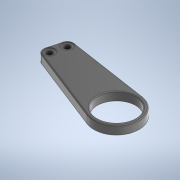
# Autodesk Inventor part: RearBumper
Saved by Autodesk Inventor 2020 (Build 240168000, 168)
## iProperties
Part Number: RearBumper
Material: PC/ABS プラスチック
Document SubType Name: Modeling
Designer: Masato Kubotera
Density: 0.357273 g/cm^3
Appearance: 滑らか - 黒
Description: TPU
Author: Masato Kubotera
Autodesk Inventor part; units mm, degrees
ref_plane "YZ Plane" through (0, 0, 0) normal (1, 0, 0) x (0, 1, 0)
ref_plane "XZ Plane" through (0, 0, 0) normal (0, 1, 0) x (-1, 0, 0)
ref_plane "XY Plane" through (0, 0, 0) normal (0, 0, 1) x (1, 0, 0)
derived "Trunk_basis.ipt"
sketch "スケッチ1" plane through (0, 0, 0) normal (0, 1, 0) x (-1, 0, 0)
  line L0 (0, 22) -> (0, -142.9) construction
  circle A0 centre (5, 0) radius 10.5 construction
  line L1 (-7, 16) -> (36, 16) construction
  line L2 (36, 16) -> (36, -16) construction
  line L3 (36, -16) -> (-7, -16) construction
  line L4 (-7, -16) -> (-7, 16) construction
  line L5 (-7, 16) -> (36, -16) construction
  line L6 (36, 16) -> (-7, -16) construction
  line L7 (33, 13.5) -> (6, 13.5) construction
  line L8 (6, 13.5) -> (6, -13.5) construction
  line L9 (6, -13.5) -> (33, -13.5) construction
  line L10 (33, -13.5) -> (33, 13.5) construction
  line L11 (33, 13.5) -> (6, -13.5) construction
  line L12 (6, 13.5) -> (33, -13.5) construction
  line L13 (-7, 0) -> (36, 0) construction
  arc A1 (5, 16) -> (-7, 10.583) centre (5, 0) ccw construction
  line L14 (43.75, -16.25) -> (5, -16.25)
  line L15 (5, 16.25) -> (43.75, 16.25)
  line L16 (44.75, 15.25) -> (44.75, -15.25)
  arc A2 (5, 16.25) -> (-6.7376, 11.2379) centre (5, 0) ccw
  arc A3 (-6.7376, 11.2379) -> (-7.25, 9.9174) centre (-6.2711, 10.2972) ccw
  circle A4 centre (6, 13.5) radius 1.35
  line L17 (19.5, 13.5) -> (19.5, -13.5) construction
  circle A5 centre (33, 13.5) radius 1.35
  line L18 (-15, 22) -> (-20, 17)
  line L19 (-20, 17) -> (-20, -19)
  line L20 (-20, -19) -> (-28.5, -27.5)
  line L21 (-28.5, -27.5) -> (-28.5, -103)
  line L22 (57.5, -22.5) -> (57.5, 17)
  line L23 (57.5, 17) -> (52.5, 22)
  line L24 (52.5, 22) -> (-15, 22)
  line L25 (-35.5597, -116.5529) -> (-28.5, -142.9)
  line L26 (-16, -139) -> (-16, -94) construction
  line L27 (-7.5, -140.4849) -> (-7.5, -142.9)
  line L28 (-7.5, -142.9) -> (7.5, -142.9)
  line L29 (7.5, -140.4849) -> (7.5, -142.9)
  arc A6 (-7.5, -140.4849) -> (-8.9849, -139) centre (-8.2425, -139.7425) ccw
  line L30 (-17.5, -138.9955) -> (-17.5, -133) construction
  line L31 (-19, -133) -> (-16, -133) construction
  line L32 (-19, -133) -> (-19, -139) construction
  line L33 (-16, -133) -> (-16, -139) construction
  line L34 (-15, 22) -> (-10, 22) construction
  line L35 (-10, 22) -> (-10, -22) construction
  line L36 (-10, -22) -> (-15, -22) construction
  line L37 (-15, -22) -> (-15, 22) construction
  line L38 (-15, 22) -> (-10, -22) construction
  line L39 (-10, 22) -> (-15, -22) construction
  line L40 (-12.5, 22) -> (-12.5, -22) construction
  line L41 (-10, 0) -> (-15, 0) construction
  circle A7 centre (-12.5, 17.75) radius 1.6
  line L42 (-15, 10) -> (-12.5, 10) construction
  line L43 (-12.5, 10) -> (-12.5, -10) construction
  line L44 (-12.5, -10) -> (-15, -10) construction
  line L45 (-15, -10) -> (-15, 10) construction
  line L46 (-15, 10) -> (-12.5, -10) construction
  line L47 (-12.5, 10) -> (-15, -10) construction
  line L48 (-12.25, 10.25) -> (-15.25, 10.25)
  line L49 (-15.25, 8.15) -> (-15.25, -8.15)
  line L50 (-15.25, -10.25) -> (-12.25, -10.25)
  line L51 (-12.25, -8.15) -> (-12.25, 8.15)
  line L52 (-12.25, 10.25) -> (-15.25, -10.25) construction
  line L53 (-15.25, 10.25) -> (-12.25, -10.25) construction
  arc A8 (-15.25, 10.25) -> (-15.25, 8.15) centre (-15.25, 9.2) ccw
  line L54 (-13.75, 10) -> (-13.75, -10) construction
  arc A9 (-12.25, 8.15) -> (-12.25, 10.25) centre (-12.25, 9.2) ccw
  circle A10 centre (-12.5, -17.75) radius 1.6
  arc A11 (-15.25, -8.15) -> (-15.25, -10.25) centre (-15.25, -9.2) ccw
  arc A12 (-12.25, -10.25) -> (-12.25, -8.15) centre (-12.25, -9.2) ccw
  line L55 (36, 14.4) -> (44.5, 14.4) construction
  line L56 (44.5, 14.4) -> (44.5, -14.4) construction
  line L57 (36, -14.4) -> (44.5, -14.4) construction
  line L58 (49.95, 7.95) -> (49.95, -7.95)
  line L59 (52.5, 0) -> (47.5, 0) construction
  line L60 (47.5, 22) -> (52.5, 22) construction
  line L61 (52.55, -7.95) -> (52.55, 7.95)
  line L62 (51.25, 10) -> (51.25, -10) construction
  line L63 (52.5, 10) -> (50, -10) construction
  line L64 (52.5, -10) -> (50, -10) construction
  line L65 (52.5, 10) -> (52.5, -10) construction
  line L66 (50, 10) -> (52.5, -10) construction
  line L67 (49.95, -10.05) -> (52.55, -10.05)
  line L68 (49.95, 10.05) -> (52.55, -10.05) construction
  line L69 (52.55, 10.05) -> (49.95, -10.05) construction
  line L70 (52.5, -22) -> (47.5, -22) construction
  line L71 (47.5, 22) -> (52.5, -22) construction
  line L72 (52.5, 22) -> (52.5, -22) construction
  line L73 (52.5, 22) -> (47.5, -22) construction
  line L74 (50, 22) -> (50, -22) construction
  line L75 (47.5, -22) -> (47.5, 22) construction
  circle A13 centre (50, -17.75) radius 1.6
  arc A14 (52.55, -10.05) -> (52.55, -7.95) centre (52.55, -9) ccw
  line L76 (50, -10) -> (50, 10) construction
  arc A15 (49.95, -7.95) -> (49.95, -10.05) centre (49.95, -9) ccw
  arc A16 (49.95, 10.05) -> (49.95, 7.95) centre (49.95, 9) ccw
  arc A17 (52.55, 7.95) -> (52.55, 10.05) centre (52.55, 9) ccw
  line L77 (50, 10) -> (52.5, 10) construction
  line L78 (52.55, 10.05) -> (49.95, 10.05)
  circle A18 centre (50, 17.75) radius 1.6
  circle A19 centre (5, 0) radius 16 construction
  arc A20 (-6.7376, -11.2379) -> (5, -16.25) centre (5, 0) ccw
  arc A21 (-7.25, -9.9174) -> (-6.7376, -11.2379) centre (-6.2711, -10.2972) ccw
  line L79 (-7.25, -9.9174) -> (-7.25, 9.9174)
  line L80 (17.5, -138.9955) -> (17.5, -133) construction
  line L81 (19, -133) -> (19, -139) construction
  line L82 (16, -133) -> (16, -139) construction
  line L83 (19, -133) -> (16, -133) construction
  circle A22 centre (6, -13.5) radius 1.35
  circle A23 centre (33, -13.5) radius 1.35
  line L84 (-25.5, -142.9) -> (-7.5, -142.9) construction
  line L85 (25.5, -142.9) -> (7.5, -142.9) construction
  line L86 (-23.5, -22.5) -> (57.5, -22.5) construction
  line L87 (57.5, -22.5) -> (57.5, -103)
  circle A24 centre (-13.5, -55) radius 1.75
  line L88 (-11.5, -59) -> (45.5, -59)
  line L89 (47.5, -61) -> (47.5, -82.5)
  line L90 (45.5, -84.5) -> (-11.5, -84.5)
  line L91 (-13.5, -82.5) -> (-13.5, -61)
  line L92 (-13.5, -59) -> (47.5, -84.5) construction
  line L93 (47.5, -59) -> (-13.5, -84.5) construction
  line L94 (-11.5, -27.5) -> (45.5, -27.5)
  line L95 (47.5, -29.5) -> (47.5, -49)
  line L96 (45.5, -51) -> (-11.5, -51)
  line L97 (-13.5, -49) -> (-13.5, -29.5)
  line L98 (-13.5, -27.5) -> (47.5, -51) construction
  line L99 (47.5, -27.5) -> (-13.5, -51) construction
  line L100 (-23.5, -108) -> (-28.5, -103)
  circle A25 centre (-20.5415, -102) radius 1.6
  line L101 (-25.7227, -96) -> (25.7227, -96)
  line L102 (25.7227, -96) -> (34.9603, -112)
  line L103 (35.5597, -116.5529) -> (28.5, -142.9)
  line L104 (-25.7227, -96) -> (-34.9603, -112)
  line L105 (57.5, -103) -> (52.5, -108)
  arc A26 (-11.5, -27.5) -> (-13.5, -29.5) centre (-11.5, -29.5) ccw
  arc A27 (-13.5, -49) -> (-11.5, -51) centre (-11.5, -49) ccw
  arc A28 (45.5, -51) -> (47.5, -49) centre (45.5, -49) ccw
  arc A29 (47.5, -29.5) -> (45.5, -27.5) centre (45.5, -29.5) ccw
  arc A30 (-11.5, -59) -> (-13.5, -61) centre (-11.5, -61) ccw
  arc A31 (-13.5, -82.5) -> (-11.5, -84.5) centre (-11.5, -82.5) ccw
  arc A32 (45.5, -84.5) -> (47.5, -82.5) centre (45.5, -82.5) ccw
  arc A33 (47.5, -61) -> (45.5, -59) centre (45.5, -61) ccw
  line L106 (-23.5, -108) -> (52.5, -108)
  line L107 (-25.5, -139) -> (-25.5, -142.9)
  line L108 (-25.5, -142.9) -> (-28.5, -142.9)
  line L109 (-17.9813, -99.3843) -> (-16.9961, -101.0907)
  line L110 (-16.9961, -102.9093) -> (-17.9813, -104.6157)
  line L111 (-19.5563, -105.525) -> (-21.5266, -105.525)
  line L112 (-23.1016, -104.6157) -> (-24.0868, -102.9093)
  line L113 (-24.0868, -101.0907) -> (-23.1016, -99.3843)
  line L114 (-21.5266, -98.475) -> (-19.5563, -98.475)
  line L115 (-16, -94) -> (16, -94) construction
  arc A34 (-24.0868, -101.0907) -> (-24.0868, -102.9093) centre (-23.5618, -102) ccw
  arc A35 (-23.1016, -104.6157) -> (-21.5266, -105.525) centre (-22.0516, -104.6157) ccw
  arc A36 (-19.5563, -105.525) -> (-17.9813, -104.6157) centre (-19.0313, -104.6157) ccw
  arc A37 (-16.9961, -102.9093) -> (-16.9961, -101.0907) centre (-17.5211, -102) ccw
  arc A38 (-17.9813, -99.3843) -> (-19.5563, -98.475) centre (-19.0313, -99.3843) ccw
  arc A39 (-21.5266, -98.475) -> (-23.1016, -99.3843) centre (-22.0516, -99.3843) ccw
  line L116 (16, -139) -> (16, -94) construction
  line L117 (16, -94) -> (-16, -94) construction
  line L118 (-25.5, -139) -> (-8.9849, -139)
  line L119 (25.5, -142.9) -> (28.5, -142.9)
  arc A40 (8.9849, -139) -> (7.5, -140.4849) centre (8.2425, -139.7425) ccw
  circle A41 centre (29.7641, -115) radius 1.25
  line L120 (33.4891, -124.2803) -> (21.898, -121.1745) construction
  line L121 (29.7641, -115) -> (25.623, -130.4548) construction
  circle A42 centre (29.7641, -115) radius 6 construction
  circle A43 centre (-20.5415, -102) radius 6 construction
  line L122 (1.9319, -109.4824) -> (7.5588, -130.4824)
  line L123 (5.6269, -133) -> (-5.6269, -133)
  line L124 (5.3151, -110.5176) -> (10.942, -131.5176)
  line L125 (12.8739, -133) -> (17.1947, -133)
  line L126 (19.1266, -131.5176) -> (24.7535, -110.5176)
  line L127 (22.8217, -108) -> (7.2469, -108)
  circle A44 centre (25.623, -130.4548) radius 1.25
  circle A45 centre (25.623, -130.4548) radius 6 construction
  line L128 (-1.9319, -109.4824) -> (-7.5588, -130.4824)
  arc A46 (1.9319, -109.4824) -> (-1.9319, -109.4824) centre (0, -110) ccw
  arc A47 (-7.5588, -130.4824) -> (-5.6269, -133) centre (-5.6269, -131) ccw
  arc A48 (5.6269, -133) -> (7.5588, -130.4824) centre (5.6269, -131) ccw
  arc A49 (7.2469, -108) -> (5.3151, -110.5176) centre (7.2469, -110) ccw
  arc A50 (24.7535, -110.5176) -> (22.8217, -108) centre (22.8217, -110) ccw
  arc A51 (17.1947, -133) -> (19.1266, -131.5176) centre (17.1947, -131) ccw
  arc A52 (10.942, -131.5176) -> (12.8739, -133) centre (12.8739, -131) ccw
  arc A53 (-5.3151, -110.5176) -> (-7.2469, -108) centre (-7.2469, -110) ccw
  line L129 (-22.8217, -108) -> (-7.2469, -108)
  line L130 (-5.3151, -110.5176) -> (-10.942, -131.5176)
  arc A54 (-22.8217, -108) -> (-24.7535, -110.5176) centre (-22.8217, -110) ccw
  line L131 (-19.1266, -131.5176) -> (-24.7535, -110.5176)
  arc A55 (-19.1266, -131.5176) -> (-17.1947, -133) centre (-17.1947, -131) ccw
  line L132 (-12.8739, -133) -> (-17.1947, -133)
  arc A56 (-12.8739, -133) -> (-10.942, -131.5176) centre (-12.8739, -131) ccw
  circle A57 centre (-29.7641, -115) radius 1.25
  circle A58 centre (-25.623, -130.4548) radius 1.25
  arc A59 (35.5597, -116.5529) -> (34.9603, -112) centre (29.7641, -115) ccw
  arc A60 (-34.9603, -112) -> (-35.5597, -116.5529) centre (-29.7641, -115) ccw
  arc A61 (-24.0151, -139) -> (-25.5, -140.4849) centre (-24.7575, -139.7425) ccw
  line L133 (25.5, -139) -> (25.5, -142.9)
  arc A62 (25.5, -140.4849) -> (24.0151, -139) centre (24.7575, -139.7425) ccw
  line L134 (25.5, -139) -> (8.9849, -139)
  line L135 (21.5266, -98.475) -> (19.5563, -98.475)
  line L136 (16.9961, -102.9093) -> (17.9813, -104.6157)
  arc A63 (21.5266, -105.525) -> (23.1016, -104.6157) centre (22.0516, -104.6157) ccw
  circle A64 centre (20.5415, -102) radius 1.6
  line L137 (24.0868, -101.0907) -> (23.1016, -99.3843)
  arc A65 (24.0868, -102.9093) -> (24.0868, -101.0907) centre (23.5618, -102) ccw
  line L138 (23.1016, -104.6157) -> (24.0868, -102.9093)
  arc A66 (23.1016, -99.3843) -> (21.5266, -98.475) centre (22.0516, -99.3843) ccw
  line L139 (19.5563, -105.525) -> (21.5266, -105.525)
  arc A67 (19.5563, -98.475) -> (17.9813, -99.3843) centre (19.0313, -99.3843) ccw
  arc A68 (17.9813, -104.6157) -> (19.5563, -105.525) centre (19.0313, -104.6157) ccw
  line L140 (17.9813, -99.3843) -> (16.9961, -101.0907)
  arc A69 (16.9961, -101.0907) -> (16.9961, -102.9093) centre (17.5211, -102) ccw
  line L141 (16, -139) -> (16, -94) construction
  circle A70 centre (20.5415, -102) radius 6 construction
  arc A71 (29.5045, -117.5445) -> (31.2612, -117.0738) centre (30.247, -116.802) ccw construction
  line L142 (31.8379, -116.4971) -> (31.2612, -117.0738) construction
  line L143 (29.5045, -117.5445) -> (28.7167, -117.3334) construction
  arc A72 (27.4307, -116.0474) -> (28.7167, -117.3334) centre (28.4449, -116.3192) ccw construction
  line L144 (27.4307, -116.0474) -> (27.2196, -115.2596) construction
  line L145 (27.6903, -113.5029) -> (28.267, -112.9262) construction
  arc A73 (30.0237, -112.4555) -> (28.267, -112.9262) centre (29.2813, -113.198) ccw construction
  arc A74 (27.6903, -113.5029) -> (27.2196, -115.2596) centre (27.9621, -114.5171) ccw construction
  line L146 (30.0237, -112.4555) -> (30.8116, -112.6666) construction
  arc A75 (31.8379, -116.4971) -> (32.3086, -114.7404) centre (31.5662, -115.4829) ccw construction
  arc A76 (32.0975, -113.9526) -> (30.8116, -112.6666) centre (31.0833, -113.6808) ccw construction
  line L147 (32.0975, -113.9526) -> (32.3086, -114.7404) construction
  line L148 (-20.5415, -102) -> (20.5415, -102) construction
  circle A77 centre (0, -102) radius 1.6
  line L149 (0.4078, -104.525) -> (-0.4078, -104.525)
  arc A78 (-0.4078, -99.475) -> (-1.9828, -100.3843) centre (-0.9328, -100.3843) ccw
  arc A79 (0.4078, -104.525) -> (1.9828, -103.6157) centre (0.9328, -103.6157) ccw
  line L150 (2.3906, -102.9093) -> (1.9828, -103.6157)
  line L151 (-0.4078, -99.475) -> (0.4078, -99.475)
  arc A80 (1.9828, -100.3843) -> (0.4078, -99.475) centre (0.9328, -100.3843) ccw
  line L152 (1.9828, -100.3843) -> (2.3906, -101.0907)
  arc A81 (2.3906, -102.9093) -> (2.3906, -101.0907) centre (1.8656, -102) ccw
  line L153 (-2.3906, -101.0907) -> (-1.9828, -100.3843)
  arc A82 (-2.3906, -101.0907) -> (-2.3906, -102.9093) centre (-1.8656, -102) ccw
  line L154 (-1.9828, -103.6157) -> (-2.3906, -102.9093)
  arc A83 (-1.9828, -103.6157) -> (-0.4078, -104.525) centre (-0.9328, -103.6157) ccw
  circle A84 centre (0, -102) radius 1.25
  arc A85 (44.75, 15.25) -> (43.75, 16.25) centre (43.75, 15.25) ccw
  arc A86 (43.75, -16.25) -> (44.75, -15.25) centre (43.75, -15.25) ccw
  circle A87 centre (-22.75, -31.75) radius 3
  circle A88 centre (-22.75, -86.75) radius 3
  line L155 (-23.5, -96) -> (-28.5, -91) construction
  line L156 (-26, -93.5) -> (-22.75, -93.5) construction
  line L157 (-26, -25) -> (-22.75, -25) construction
  line L158 (-26, -25) -> (-26, -93.5) construction
  line L159 (-22.75, -25) -> (-22.75, -93.5) construction
  line L160 (-22.75, -59.25) -> (-28.5, -59.25) construction
  point P0 (0, 0)
  point P1 (14.5, 0)
  point P2 (19.5, 0)
  point P3 (44.75, 16.25)
  point P4 (-7.25, 10.6771)
  point P5 (19.5, 0)
  point P6 (-12.5, 0)
  point P7 (-13.75, 0)
  point P8 (44.75, 14.4)
  point P9 (44.75, -14.4)
  point P10 (51.25, 0)
  point P11 (50, 0)
  point P12 (44.75, -16.25)
  point P13 (17, -71.75)
  point P14 (17, -39.25)
  point P15 (-18.5063, -98.475)
  point P16 (-16.4711, -102)
  point P17 (-18.5063, -105.525)
  point P18 (-22.5766, -105.525)
  point P19 (-22.5766, -98.475)
  point P20 (-24.6118, -102)
  point P21 (-22.5766, -105.525)
  point P22 (-18.5063, -105.525)
  point P23 (-16.4711, -102)
  point P24 (-18.5063, -98.475)
  point P25 (-22.5766, -98.475)
  point P26 (27.6936, -122.7274)
  point P27 (0, -102.2726)
  point P28 (0, -133)
  point P29 (-7.5, -139)
  point P30 (-22.5766, -98.475)
  point P31 (18.5063, -98.475)
  point P32 (18.5063, -98.475)
  point P33 (22.5766, -105.525)
  point P34 (22.5766, -105.525)
  point P35 (24.6118, -102)
  point P36 (22.5766, -98.475)
  point P37 (22.5766, -98.475)
  point P38 (22.5766, -98.475)
  point P39 (18.5063, -105.525)
  point P40 (16.4711, -102)
  point P41 (16.4711, -102)
  point P42 (18.5063, -105.525)
  point P43 (29.7641, -115)
  point P44 (29.7641, -115)
  point P45 (30.5187, -117.8163)
  point P46 (30.5187, -117.8163)
  point P47 (27.7025, -117.0617)
  point P48 (27.7025, -117.0617)
  point P49 (31.8258, -112.9383)
  point P50 (26.9479, -114.2454)
  point P51 (29.0095, -112.1837)
  point P52 (29.0095, -112.1837)
  point P53 (31.8258, -112.9383)
  point P54 (29.0095, -112.1837)
  point P55 (32.5804, -115.7546)
  point P56 (-1.4578, -99.475)
  point P57 (-1.4578, -99.475)
  point P58 (-1.4578, -99.475)
  point P59 (1.4578, -104.525)
  point P60 (1.4578, -99.475)
  point P61 (1.4578, -99.475)
  point P62 (2.9156, -102)
  point P63 (-2.9156, -102)
  point P64 (-1.4578, -104.525)
  point P65 (-1.4578, -104.525)
sketch "スケッチ2" plane through (0, 0, 0) normal (0, 1, 0) x (-1, 0, 0)
  circle A0 centre (29.7641, -115) radius 1.25 projected
  circle A1 centre (25.623, -130.4548) radius 1.25 projected
  circle A2 centre (29.7641, -115) radius 3.25
  arc A3 (30.8128, -108.079) -> (23.0026, -113.1883) centre (29.7641, -115) ccw
  line L0 (30.8128, -108.079) -> (118.7454, -121.4033)
  line L1 (33.4891, -124.2803) -> (21.898, -121.1745) construction
  circle A4 centre (25.623, -130.4548) radius 3.25
  arc A5 (18.8615, -128.6431) -> (23.0707, -136.9729) centre (25.623, -130.4548) ccw
  line L2 (23.0707, -136.9729) -> (105.8847, -169.4001)
  line L3 (0, 22) -> (0, -142.9) construction
  line L4 (23.0026, -113.1883) -> (18.8615, -128.6431)
  circle A6 centre (29.7641, -115) radius 6
  circle A7 centre (25.623, -130.4548) radius 6
  arc A8 (105.8847, -169.4001) -> (118.7454, -121.4033) centre (115, -146.1211) ccw
  circle A9 centre (115, -146.1211) radius 21
  point P0 (0, 0)
  dimension "d1" = 6.5
  dimension "d2" = 7
  dimension "d6" = 12
  dimension "d130" = 4
  dimension "d131" = 115
  dimension "d132" = 50
  constraints: 8 centre point, 6 end point, 6 point on circle, 5 coincident, 5 symmetric about line, 4 tangent, 4 other
  measures "d1" diameter of A2
  measures "d2" radius of A3
  measures "d6" diameter of A6
  measures "d130" radial gap between concentric circles of A8 A9
  measures "d131" distance from line of A8.centre L3
  measures "d132" diameter of A8
extrude "押し出し1" add sketch "スケッチ2" along normal blind 10 contours L0 A8 L2 A5 L4 A3
extrude "押し出し2" add sketch "スケッチ2" along normal blind 9 contours A6 | A7
fillet "フィレット1" radius 1 14 edges at (-25.932, 0, -109.1421) (-20.9321, 0, -120.9157) (-19.3754, 0, -133.6118) (-64.4777, 0, -153.1865) (-74.7791, 0, -114.7411) (-25.932, 10, -109.1421) (-20.9321, 10, -120.9157) (-19.3754, 10, -133.6118) (-64.4777, 10, -153.1865) (-74.7791, 10, -114.7411) (-139.1481, 10, -152.5916) (-139.1481, 0, -152.5916) (-94, 10, -146.1211) (-94, 0, -146.1211)
